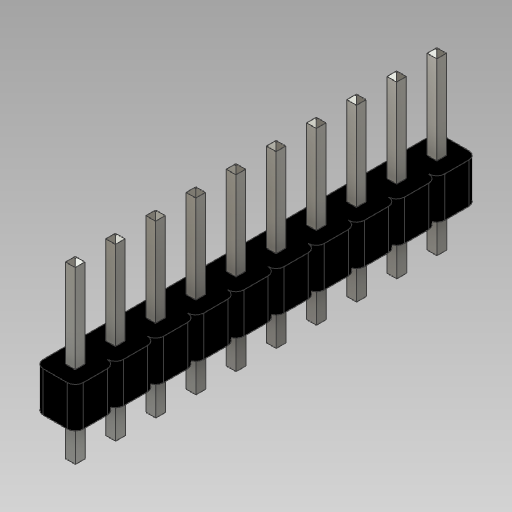
# Autodesk Inventor part: 10 pin header
Saved by Autodesk Inventor 2020 (Build 240168000, 168)
## iProperties
Created: 2017-07-30
Part Number: 10 pin header
Material: Generic
Document SubType Name: Modeling
Designer: Alex
Density: 1 g/cm^3
Appearance: Default
Author: Alex
Autodesk Inventor part; units mm, degrees
ref_plane "YZ Plane" through (0, 0, 0) normal (1, 0, 0) x (0, 1, 0)
ref_plane "XZ Plane" through (0, 0, 0) normal (0, 1, 0) x (-1, 0, 0)
ref_plane "XY Plane" through (0, 0, 0) normal (0, 0, 1) x (1, 0, 0)
sketch "Sketch1" plane through (0, 0, 0) normal (0, 1, 0) x (-1, 0, 0)
  line L0 (-0.762, -1.27) -> (0.762, -1.27)
  line L1 (1.27, -0.762) -> (1.27, 0.762)
  line L2 (0.762, 1.27) -> (-0.762, 1.27)
  line L3 (-1.27, 0.762) -> (-1.27, -0.762)
  line L4 (-1.27, -1.27) -> (1.27, 1.27) construction
  line L5 (1.27, -1.27) -> (-1.27, 1.27) construction
  arc A0 (1.27, 0.762) -> (0.762, 1.27) centre (0.762, 0.762) ccw
  arc A1 (0.762, -1.27) -> (1.27, -0.762) centre (0.762, -0.762) ccw
  arc A2 (-1.27, -0.762) -> (-0.762, -1.27) centre (-0.762, -0.762) ccw
  arc A3 (-0.762, 1.27) -> (-1.27, 0.762) centre (-0.762, 0.762) ccw
  line L6 (-0.762, -3.81) -> (0.762, -3.81)
  line L7 (1.27, -3.302) -> (1.27, -1.778)
  line L8 (0.762, -1.27) -> (-0.762, -1.27)
  line L9 (-1.27, -1.778) -> (-1.27, -3.302)
  line L10 (-1.27, -3.81) -> (1.27, -1.27) construction
  line L11 (1.27, -3.81) -> (-1.27, -1.27) construction
  arc A4 (1.27, -1.778) -> (0.762, -1.27) centre (0.762, -1.778) ccw
  arc A5 (0.762, -3.81) -> (1.27, -3.302) centre (0.762, -3.302) ccw
  arc A6 (-1.27, -3.302) -> (-0.762, -3.81) centre (-0.762, -3.302) ccw
  arc A7 (-0.762, -1.27) -> (-1.27, -1.778) centre (-0.762, -1.778) ccw
  line L12 (-0.762, -6.35) -> (0.762, -6.35)
  line L13 (1.27, -5.842) -> (1.27, -4.318)
  line L14 (0.762, -3.81) -> (-0.762, -3.81)
  line L15 (-1.27, -4.318) -> (-1.27, -5.842)
  line L16 (-1.27, -6.35) -> (1.27, -3.81) construction
  line L17 (1.27, -6.35) -> (-1.27, -3.81) construction
  arc A8 (1.27, -4.318) -> (0.762, -3.81) centre (0.762, -4.318) ccw
  arc A9 (0.762, -6.35) -> (1.27, -5.842) centre (0.762, -5.842) ccw
  arc A10 (-1.27, -5.842) -> (-0.762, -6.35) centre (-0.762, -5.842) ccw
  arc A11 (-0.762, -3.81) -> (-1.27, -4.318) centre (-0.762, -4.318) ccw
  line L18 (-0.762, -8.89) -> (0.762, -8.89)
  line L19 (1.27, -8.382) -> (1.27, -6.858)
  line L20 (0.762, -6.35) -> (-0.762, -6.35)
  line L21 (-1.27, -6.858) -> (-1.27, -8.382)
  line L22 (-1.27, -8.89) -> (1.27, -6.35) construction
  line L23 (1.27, -8.89) -> (-1.27, -6.35) construction
  arc A12 (1.27, -6.858) -> (0.762, -6.35) centre (0.762, -6.858) ccw
  arc A13 (0.762, -8.89) -> (1.27, -8.382) centre (0.762, -8.382) ccw
  arc A14 (-1.27, -8.382) -> (-0.762, -8.89) centre (-0.762, -8.382) ccw
  arc A15 (-0.762, -6.35) -> (-1.27, -6.858) centre (-0.762, -6.858) ccw
  line L24 (-0.762, -11.43) -> (0.762, -11.43)
  line L25 (1.27, -10.922) -> (1.27, -9.398)
  line L26 (0.762, -8.89) -> (-0.762, -8.89)
  line L27 (-1.27, -9.398) -> (-1.27, -10.922)
  line L28 (-1.27, -11.43) -> (1.27, -8.89) construction
  line L29 (1.27, -11.43) -> (-1.27, -8.89) construction
  arc A16 (1.27, -9.398) -> (0.762, -8.89) centre (0.762, -9.398) ccw
  arc A17 (0.762, -11.43) -> (1.27, -10.922) centre (0.762, -10.922) ccw
  arc A18 (-1.27, -10.922) -> (-0.762, -11.43) centre (-0.762, -10.922) ccw
  arc A19 (-0.762, -8.89) -> (-1.27, -9.398) centre (-0.762, -9.398) ccw
  line L30 (-0.762, -13.97) -> (0.762, -13.97)
  line L31 (1.27, -13.462) -> (1.27, -11.938)
  line L32 (0.762, -11.43) -> (-0.762, -11.43)
  line L33 (-1.27, -11.938) -> (-1.27, -13.462)
  line L34 (-1.27, -13.97) -> (1.27, -11.43) construction
  line L35 (1.27, -13.97) -> (-1.27, -11.43) construction
  arc A20 (1.27, -11.938) -> (0.762, -11.43) centre (0.762, -11.938) ccw
  arc A21 (0.762, -13.97) -> (1.27, -13.462) centre (0.762, -13.462) ccw
  arc A22 (-1.27, -13.462) -> (-0.762, -13.97) centre (-0.762, -13.462) ccw
  arc A23 (-0.762, -11.43) -> (-1.27, -11.938) centre (-0.762, -11.938) ccw
  line L36 (-0.762, -16.51) -> (0.762, -16.51)
  line L37 (1.27, -16.002) -> (1.27, -14.478)
  line L38 (0.762, -13.97) -> (-0.762, -13.97)
  line L39 (-1.27, -14.478) -> (-1.27, -16.002)
  line L40 (-1.27, -16.51) -> (1.27, -13.97) construction
  line L41 (1.27, -16.51) -> (-1.27, -13.97) construction
  arc A24 (1.27, -14.478) -> (0.762, -13.97) centre (0.762, -14.478) ccw
  arc A25 (0.762, -16.51) -> (1.27, -16.002) centre (0.762, -16.002) ccw
  arc A26 (-1.27, -16.002) -> (-0.762, -16.51) centre (-0.762, -16.002) ccw
  arc A27 (-0.762, -13.97) -> (-1.27, -14.478) centre (-0.762, -14.478) ccw
  line L42 (-0.762, -19.05) -> (0.762, -19.05)
  line L43 (1.27, -18.542) -> (1.27, -17.018)
  line L44 (0.762, -16.51) -> (-0.762, -16.51)
  line L45 (-1.27, -17.018) -> (-1.27, -18.542)
  line L46 (-1.27, -19.05) -> (1.27, -16.51) construction
  line L47 (1.27, -19.05) -> (-1.27, -16.51) construction
  arc A28 (1.27, -17.018) -> (0.762, -16.51) centre (0.762, -17.018) ccw
  arc A29 (0.762, -19.05) -> (1.27, -18.542) centre (0.762, -18.542) ccw
  arc A30 (-1.27, -18.542) -> (-0.762, -19.05) centre (-0.762, -18.542) ccw
  arc A31 (-0.762, -16.51) -> (-1.27, -17.018) centre (-0.762, -17.018) ccw
  line L48 (-0.762, -21.59) -> (0.762, -21.59)
  line L49 (1.27, -21.082) -> (1.27, -19.558)
  line L50 (0.762, -19.05) -> (-0.762, -19.05)
  line L51 (-1.27, -19.558) -> (-1.27, -21.082)
  line L52 (-1.27, -21.59) -> (1.27, -19.05) construction
  line L53 (1.27, -21.59) -> (-1.27, -19.05) construction
  arc A32 (1.27, -19.558) -> (0.762, -19.05) centre (0.762, -19.558) ccw
  arc A33 (0.762, -21.59) -> (1.27, -21.082) centre (0.762, -21.082) ccw
  arc A34 (-1.27, -21.082) -> (-0.762, -21.59) centre (-0.762, -21.082) ccw
  arc A35 (-0.762, -19.05) -> (-1.27, -19.558) centre (-0.762, -19.558) ccw
  line L54 (-0.762, -24.13) -> (0.762, -24.13)
  line L55 (1.27, -23.622) -> (1.27, -22.098)
  line L56 (0.762, -21.59) -> (-0.762, -21.59)
  line L57 (-1.27, -22.098) -> (-1.27, -23.622)
  line L58 (-1.27, -24.13) -> (1.27, -21.59) construction
  line L59 (1.27, -24.13) -> (-1.27, -21.59) construction
  arc A36 (1.27, -22.098) -> (0.762, -21.59) centre (0.762, -22.098) ccw
  arc A37 (0.762, -24.13) -> (1.27, -23.622) centre (0.762, -23.622) ccw
  arc A38 (-1.27, -23.622) -> (-0.762, -24.13) centre (-0.762, -23.622) ccw
  arc A39 (-0.762, -21.59) -> (-1.27, -22.098) centre (-0.762, -22.098) ccw
  line L60 (-0.762, -26.67) -> (0.762, -26.67)
  line L61 (1.27, -26.162) -> (1.27, -24.638)
  line L62 (0.762, -24.13) -> (-0.762, -24.13)
  line L63 (-1.27, -24.638) -> (-1.27, -26.162)
  line L64 (-1.27, -26.67) -> (1.27, -24.13) construction
  line L65 (1.27, -26.67) -> (-1.27, -24.13) construction
  arc A40 (1.27, -24.638) -> (0.762, -24.13) centre (0.762, -24.638) ccw
  arc A41 (0.762, -26.67) -> (1.27, -26.162) centre (0.762, -26.162) ccw
  arc A42 (-1.27, -26.162) -> (-0.762, -26.67) centre (-0.762, -26.162) ccw
  arc A43 (-0.762, -24.13) -> (-1.27, -24.638) centre (-0.762, -24.638) ccw
  line L66 (-0.762, -29.21) -> (0.762, -29.21)
  line L67 (1.27, -28.702) -> (1.27, -27.178)
  line L68 (0.762, -26.67) -> (-0.762, -26.67)
  line L69 (-1.27, -27.178) -> (-1.27, -28.702)
  line L70 (-1.27, -29.21) -> (1.27, -26.67) construction
  line L71 (1.27, -29.21) -> (-1.27, -26.67) construction
  arc A44 (1.27, -27.178) -> (0.762, -26.67) centre (0.762, -27.178) ccw
  arc A45 (0.762, -29.21) -> (1.27, -28.702) centre (0.762, -28.702) ccw
  arc A46 (-1.27, -28.702) -> (-0.762, -29.21) centre (-0.762, -28.702) ccw
  arc A47 (-0.762, -26.67) -> (-1.27, -27.178) centre (-0.762, -27.178) ccw
  line L72 (-0.762, -31.75) -> (0.762, -31.75)
  line L73 (1.27, -31.242) -> (1.27, -29.718)
  line L74 (0.762, -29.21) -> (-0.762, -29.21)
  line L75 (-1.27, -29.718) -> (-1.27, -31.242)
  line L76 (-1.27, -31.75) -> (1.27, -29.21) construction
  line L77 (1.27, -31.75) -> (-1.27, -29.21) construction
  arc A48 (1.27, -29.718) -> (0.762, -29.21) centre (0.762, -29.718) ccw
  arc A49 (0.762, -31.75) -> (1.27, -31.242) centre (0.762, -31.242) ccw
  arc A50 (-1.27, -31.242) -> (-0.762, -31.75) centre (-0.762, -31.242) ccw
  arc A51 (-0.762, -29.21) -> (-1.27, -29.718) centre (-0.762, -29.718) ccw
  line L78 (-0.762, -34.29) -> (0.762, -34.29)
  line L79 (1.27, -33.782) -> (1.27, -32.258)
  line L80 (0.762, -31.75) -> (-0.762, -31.75)
  line L81 (-1.27, -32.258) -> (-1.27, -33.782)
  line L82 (-1.27, -34.29) -> (1.27, -31.75) construction
  line L83 (1.27, -34.29) -> (-1.27, -31.75) construction
  arc A52 (1.27, -32.258) -> (0.762, -31.75) centre (0.762, -32.258) ccw
  arc A53 (0.762, -34.29) -> (1.27, -33.782) centre (0.762, -33.782) ccw
  arc A54 (-1.27, -33.782) -> (-0.762, -34.29) centre (-0.762, -33.782) ccw
  arc A55 (-0.762, -31.75) -> (-1.27, -32.258) centre (-0.762, -32.258) ccw
  line L84 (-0.762, -36.83) -> (0.762, -36.83)
  line L85 (1.27, -36.322) -> (1.27, -34.798)
  line L86 (0.762, -34.29) -> (-0.762, -34.29)
  line L87 (-1.27, -34.798) -> (-1.27, -36.322)
  line L88 (-1.27, -36.83) -> (1.27, -34.29) construction
  line L89 (1.27, -36.83) -> (-1.27, -34.29) construction
  arc A56 (1.27, -34.798) -> (0.762, -34.29) centre (0.762, -34.798) ccw
  arc A57 (0.762, -36.83) -> (1.27, -36.322) centre (0.762, -36.322) ccw
  arc A58 (-1.27, -36.322) -> (-0.762, -36.83) centre (-0.762, -36.322) ccw
  arc A59 (-0.762, -34.29) -> (-1.27, -34.798) centre (-0.762, -34.798) ccw
  line L90 (-0.762, -39.37) -> (0.762, -39.37)
  line L91 (1.27, -38.862) -> (1.27, -37.338)
  line L92 (0.762, -36.83) -> (-0.762, -36.83)
  line L93 (-1.27, -37.338) -> (-1.27, -38.862)
  line L94 (-1.27, -39.37) -> (1.27, -36.83) construction
  line L95 (1.27, -39.37) -> (-1.27, -36.83) construction
  arc A60 (1.27, -37.338) -> (0.762, -36.83) centre (0.762, -37.338) ccw
  arc A61 (0.762, -39.37) -> (1.27, -38.862) centre (0.762, -38.862) ccw
  arc A62 (-1.27, -38.862) -> (-0.762, -39.37) centre (-0.762, -38.862) ccw
  arc A63 (-0.762, -36.83) -> (-1.27, -37.338) centre (-0.762, -37.338) ccw
  point P0 (0, 0)
  point P1 (0, -2.54)
  point P2 (0, -5.08)
  point P3 (0, -7.62)
  point P4 (0, -10.16)
  point P5 (0, -12.7)
  point P6 (0, -15.24)
  point P7 (0, -17.78)
  point P8 (0, -20.32)
  point P9 (0, -22.86)
  point P10 (0, -25.4)
  point P11 (0, -27.94)
  point P12 (0, -30.48)
  point P13 (0, -33.02)
  point P14 (0, -35.56)
  point P15 (0, -38.1)
  dimension "d0" = 2.54
  dimension "d1" = 0.508
  dimension "d4" = 2.54
  constraints: 192 end point, 128 point on circle, 128 point on line, 64 centre point, 32 midpoint, 8 tangent, 3 equal radius, 2 parallel, 2 perpendicular, 1 collinear, 1 horizontal, 1 vertical, 404 other
  measures "d0" distance between parallel lines of L0 L2
  measures "d1" radius of A0
  measures "d4" distance of point (0, 0) point (0, -2.54)
extrude "Extrusion1" add sketch "Sketch1" along normal mid plane 2.54
sketch "Sketch2" plane through (0, 1.27, 0) normal (0, 1, 0) x (1, 0, 0)
  line L0 (-0.3048, 0.3048) -> (0.3048, 0.3048)
  line L1 (0.3048, 0.3048) -> (0.3048, -0.3048)
  line L2 (0.3048, -0.3048) -> (-0.3048, -0.3048)
  line L3 (-0.3048, -0.3048) -> (-0.3048, 0.3048)
  line L4 (-0.3048, 0.3048) -> (0.3048, -0.3048) construction
  line L5 (0.3048, 0.3048) -> (-0.3048, -0.3048) construction
  line L6 (-1.27, 0.762) -> (-1.27, -0.762) projected
  line L7 (-0.3048, 2.8448) -> (0.3048, 2.8448)
  line L8 (0.3048, 2.8448) -> (0.3048, 2.2352)
  line L9 (0.3048, 2.2352) -> (-0.3048, 2.2352)
  line L10 (-0.3048, 2.2352) -> (-0.3048, 2.8448)
  line L11 (-0.3048, 2.8448) -> (0.3048, 2.2352) construction
  line L12 (0.3048, 2.8448) -> (-0.3048, 2.2352) construction
  line L13 (-0.3048, 5.3848) -> (0.3048, 5.3848)
  line L14 (0.3048, 5.3848) -> (0.3048, 4.7752)
  line L15 (0.3048, 4.7752) -> (-0.3048, 4.7752)
  line L16 (-0.3048, 4.7752) -> (-0.3048, 5.3848)
  line L17 (-0.3048, 5.3848) -> (0.3048, 4.7752) construction
  line L18 (0.3048, 5.3848) -> (-0.3048, 4.7752) construction
  line L19 (-0.3048, 7.9248) -> (0.3048, 7.9248)
  line L20 (0.3048, 7.9248) -> (0.3048, 7.3152)
  line L21 (0.3048, 7.3152) -> (-0.3048, 7.3152)
  line L22 (-0.3048, 7.3152) -> (-0.3048, 7.9248)
  line L23 (-0.3048, 7.9248) -> (0.3048, 7.3152) construction
  line L24 (0.3048, 7.9248) -> (-0.3048, 7.3152) construction
  line L25 (-0.3048, 10.4648) -> (0.3048, 10.4648)
  line L26 (0.3048, 10.4648) -> (0.3048, 9.8552)
  line L27 (0.3048, 9.8552) -> (-0.3048, 9.8552)
  line L28 (-0.3048, 9.8552) -> (-0.3048, 10.4648)
  line L29 (-0.3048, 10.4648) -> (0.3048, 9.8552) construction
  line L30 (0.3048, 10.4648) -> (-0.3048, 9.8552) construction
  line L31 (-0.3048, 13.0048) -> (0.3048, 13.0048)
  line L32 (0.3048, 13.0048) -> (0.3048, 12.3952)
  line L33 (0.3048, 12.3952) -> (-0.3048, 12.3952)
  line L34 (-0.3048, 12.3952) -> (-0.3048, 13.0048)
  line L35 (-0.3048, 13.0048) -> (0.3048, 12.3952) construction
  line L36 (0.3048, 13.0048) -> (-0.3048, 12.3952) construction
  line L37 (-0.3048, 15.5448) -> (0.3048, 15.5448)
  line L38 (0.3048, 15.5448) -> (0.3048, 14.9352)
  line L39 (0.3048, 14.9352) -> (-0.3048, 14.9352)
  line L40 (-0.3048, 14.9352) -> (-0.3048, 15.5448)
  line L41 (-0.3048, 15.5448) -> (0.3048, 14.9352) construction
  line L42 (0.3048, 15.5448) -> (-0.3048, 14.9352) construction
  line L43 (-0.3048, 18.0848) -> (0.3048, 18.0848)
  line L44 (0.3048, 18.0848) -> (0.3048, 17.4752)
  line L45 (0.3048, 17.4752) -> (-0.3048, 17.4752)
  line L46 (-0.3048, 17.4752) -> (-0.3048, 18.0848)
  line L47 (-0.3048, 18.0848) -> (0.3048, 17.4752) construction
  line L48 (0.3048, 18.0848) -> (-0.3048, 17.4752) construction
  line L49 (-0.3048, 20.6248) -> (0.3048, 20.6248)
  line L50 (0.3048, 20.6248) -> (0.3048, 20.0152)
  line L51 (0.3048, 20.0152) -> (-0.3048, 20.0152)
  line L52 (-0.3048, 20.0152) -> (-0.3048, 20.6248)
  line L53 (-0.3048, 20.6248) -> (0.3048, 20.0152) construction
  line L54 (0.3048, 20.6248) -> (-0.3048, 20.0152) construction
  line L55 (-0.3048, 23.1648) -> (0.3048, 23.1648)
  line L56 (0.3048, 23.1648) -> (0.3048, 22.5552)
  line L57 (0.3048, 22.5552) -> (-0.3048, 22.5552)
  line L58 (-0.3048, 22.5552) -> (-0.3048, 23.1648)
  line L59 (-0.3048, 23.1648) -> (0.3048, 22.5552) construction
  line L60 (0.3048, 23.1648) -> (-0.3048, 22.5552) construction
  line L61 (-0.3048, 25.7048) -> (0.3048, 25.7048)
  line L62 (0.3048, 25.7048) -> (0.3048, 25.0952)
  line L63 (0.3048, 25.0952) -> (-0.3048, 25.0952)
  line L64 (-0.3048, 25.0952) -> (-0.3048, 25.7048)
  line L65 (-0.3048, 25.7048) -> (0.3048, 25.0952) construction
  line L66 (0.3048, 25.7048) -> (-0.3048, 25.0952) construction
  line L67 (-0.3048, 28.2448) -> (0.3048, 28.2448)
  line L68 (0.3048, 28.2448) -> (0.3048, 27.6352)
  line L69 (0.3048, 27.6352) -> (-0.3048, 27.6352)
  line L70 (-0.3048, 27.6352) -> (-0.3048, 28.2448)
  line L71 (-0.3048, 28.2448) -> (0.3048, 27.6352) construction
  line L72 (0.3048, 28.2448) -> (-0.3048, 27.6352) construction
  line L73 (-0.3048, 30.7848) -> (0.3048, 30.7848)
  line L74 (0.3048, 30.7848) -> (0.3048, 30.1752)
  line L75 (0.3048, 30.1752) -> (-0.3048, 30.1752)
  line L76 (-0.3048, 30.1752) -> (-0.3048, 30.7848)
  line L77 (-0.3048, 30.7848) -> (0.3048, 30.1752) construction
  line L78 (0.3048, 30.7848) -> (-0.3048, 30.1752) construction
  line L79 (-0.3048, 33.3248) -> (0.3048, 33.3248)
  line L80 (0.3048, 33.3248) -> (0.3048, 32.7152)
  line L81 (0.3048, 32.7152) -> (-0.3048, 32.7152)
  line L82 (-0.3048, 32.7152) -> (-0.3048, 33.3248)
  line L83 (-0.3048, 33.3248) -> (0.3048, 32.7152) construction
  line L84 (0.3048, 33.3248) -> (-0.3048, 32.7152) construction
  line L85 (-0.3048, 35.8648) -> (0.3048, 35.8648)
  line L86 (0.3048, 35.8648) -> (0.3048, 35.2552)
  line L87 (0.3048, 35.2552) -> (-0.3048, 35.2552)
  line L88 (-0.3048, 35.2552) -> (-0.3048, 35.8648)
  line L89 (-0.3048, 35.8648) -> (0.3048, 35.2552) construction
  line L90 (0.3048, 35.8648) -> (-0.3048, 35.2552) construction
  line L91 (-0.3048, 38.4048) -> (0.3048, 38.4048)
  line L92 (0.3048, 38.4048) -> (0.3048, 37.7952)
  line L93 (0.3048, 37.7952) -> (-0.3048, 37.7952)
  line L94 (-0.3048, 37.7952) -> (-0.3048, 38.4048)
  line L95 (-0.3048, 38.4048) -> (0.3048, 37.7952) construction
  line L96 (0.3048, 38.4048) -> (-0.3048, 37.7952) construction
  point P0 (0, 0)
  dimension "d11" = 0.6096
  dimension "d14" = 2.54
  constraints: 192 end point, 2 midpoint, 2 parallel, 2 perpendicular, 1 horizontal, 1 vertical, 150 other
  measures "d11" distance of L2.end L0.start
  measures "d14" distance of L0.start L7.start
extrude "Extrusion2" add sketch "Sketch2" along normal blind 5.842
chamfer "Chamfer2" distance 0.254 angle 45 64 edges at (0, 7.112, -20.6248) (-0.3048, 7.112, -20.32) (0.3048, 7.112, -20.32) (0, 7.112, -20.0152) (0, 7.112, -18.0848) (-0.3048, 7.112, -17.78) (0, 7.112, -17.4752) (0.3048, 7.112, -17.78) (0, 7.112, -15.5448) (-0.3048, 7.112, -15.24) (0.3048, 7.112, -15.24) (0, 7.112, -13.0048) (-0.3048, 7.112, -12.7) (0, 7.112, -12.3952) (0.3048, 7.112, -12.7) (0, 7.112, -14.9352) (-0.3048, 7.112, -7.62) (0, 7.112, -7.3152) (0.3048, 7.112, -7.62) (0, 7.112, -9.8552) (0, 7.112, -10.4648) (-0.3048, 7.112, -10.16) (0.3048, 7.112, -10.16) (0, 7.112, -7.9248) (0, 7.112, -2.8448) (-0.3048, 7.112, -2.54) (0, 7.112, -2.2352) (0.3048, 7.112, -2.54) (0, 7.112, -4.7752) (0.3048, 7.112, -5.08) (0, 7.112, -5.3848) (-0.3048, 7.112, -5.08) (0, 7.112, -0.3048) (-0.3048, 7.112, 0) (0, 7.112, 0.3048) (0.3048, 7.112, 0) (0, 7.112, -23.1648) (-0.3048, 7.112, -22.86) (0, 7.112, -22.5552) (0.3048, 7.112, -22.86) (0, 7.112, -25.0952) (-0.3048, 7.112, -25.4) (0, 7.112, -25.7048) (0.3048, 7.112, -25.4) (0, 7.112, -28.2448) (0, 7.112, -27.6352) (0.3048, 7.112, -27.94) (-0.3048, 7.112, -27.94) (0.3048, 7.112, -30.48) (0, 7.112, -38.4048) (-0.3048, 7.112, -38.1) (0, 7.112, -37.7952) (0.3048, 7.112, -38.1) (0, 7.112, -35.8648) (-0.3048, 7.112, -35.56) (0, 7.112, -35.2552) (0.3048, 7.112, -35.56) (0, 7.112, -33.3248) (-0.3048, 7.112, -33.02) (0, 7.112, -32.7152) (0, 7.112, -30.1752) (0, 7.112, -30.7848) (-0.3048, 7.112, -30.48) (0.3048, 7.112, -33.02)
sketch "Sketch6" plane through (0, -1.27, 0) normal (0, -1, 0) x (1, 0, 0)
  line L0 (-0.3048, 0.3048) -> (-0.3048, -0.3048) projected
  line L1 (0.3175, -0.3175) -> (-0.3048, -0.3175)
  line L2 (-0.3048, -0.3175) -> (-0.3048, 0.3048)
  line L3 (-0.3048, 0.3048) -> (0.3175, 0.3048)
  line L4 (0.3175, 0.3048) -> (0.3175, -0.3175)
  line L5 (0.3175, -0.3175) -> (-0.3048, 0.3048) construction
  line L6 (-0.3048, -0.3175) -> (0.3175, 0.3048) construction
  line L7 (1.27, -0.762) -> (1.27, 0.762) construction
  line L8 (0.3175, -2.8575) -> (-0.3048, -2.8575)
  line L9 (-0.3048, -2.8575) -> (-0.3048, -2.2352)
  line L10 (-0.3048, -2.2352) -> (0.3175, -2.2352)
  line L11 (0.3175, -2.2352) -> (0.3175, -2.8575)
  line L12 (0.3175, -2.8575) -> (-0.3048, -2.2352) construction
  line L13 (-0.3048, -2.8575) -> (0.3175, -2.2352) construction
  line L14 (0.3175, -5.3975) -> (-0.3048, -5.3975)
  line L15 (-0.3048, -5.3975) -> (-0.3048, -4.7752)
  line L16 (-0.3048, -4.7752) -> (0.3175, -4.7752)
  line L17 (0.3175, -4.7752) -> (0.3175, -5.3975)
  line L18 (0.3175, -5.3975) -> (-0.3048, -4.7752) construction
  line L19 (-0.3048, -5.3975) -> (0.3175, -4.7752) construction
  line L20 (0.3175, -7.9375) -> (-0.3048, -7.9375)
  line L21 (-0.3048, -7.9375) -> (-0.3048, -7.3152)
  line L22 (-0.3048, -7.3152) -> (0.3175, -7.3152)
  line L23 (0.3175, -7.3152) -> (0.3175, -7.9375)
  line L24 (0.3175, -7.9375) -> (-0.3048, -7.3152) construction
  line L25 (-0.3048, -7.9375) -> (0.3175, -7.3152) construction
  line L26 (0.3175, -10.4775) -> (-0.3048, -10.4775)
  line L27 (-0.3048, -10.4775) -> (-0.3048, -9.8552)
  line L28 (-0.3048, -9.8552) -> (0.3175, -9.8552)
  line L29 (0.3175, -9.8552) -> (0.3175, -10.4775)
  line L30 (0.3175, -10.4775) -> (-0.3048, -9.8552) construction
  line L31 (-0.3048, -10.4775) -> (0.3175, -9.8552) construction
  line L32 (0.3175, -13.0175) -> (-0.3048, -13.0175)
  line L33 (-0.3048, -13.0175) -> (-0.3048, -12.3952)
  line L34 (-0.3048, -12.3952) -> (0.3175, -12.3952)
  line L35 (0.3175, -12.3952) -> (0.3175, -13.0175)
  line L36 (0.3175, -13.0175) -> (-0.3048, -12.3952) construction
  line L37 (-0.3048, -13.0175) -> (0.3175, -12.3952) construction
  line L38 (0.3175, -15.5575) -> (-0.3048, -15.5575)
  line L39 (-0.3048, -15.5575) -> (-0.3048, -14.9352)
  line L40 (-0.3048, -14.9352) -> (0.3175, -14.9352)
  line L41 (0.3175, -14.9352) -> (0.3175, -15.5575)
  line L42 (0.3175, -15.5575) -> (-0.3048, -14.9352) construction
  line L43 (-0.3048, -15.5575) -> (0.3175, -14.9352) construction
  line L44 (0.3175, -18.0975) -> (-0.3048, -18.0975)
  line L45 (-0.3048, -18.0975) -> (-0.3048, -17.4752)
  line L46 (-0.3048, -17.4752) -> (0.3175, -17.4752)
  line L47 (0.3175, -17.4752) -> (0.3175, -18.0975)
  line L48 (0.3175, -18.0975) -> (-0.3048, -17.4752) construction
  line L49 (-0.3048, -18.0975) -> (0.3175, -17.4752) construction
  line L50 (0.3175, -20.6375) -> (-0.3048, -20.6375)
  line L51 (-0.3048, -20.6375) -> (-0.3048, -20.0152)
  line L52 (-0.3048, -20.0152) -> (0.3175, -20.0152)
  line L53 (0.3175, -20.0152) -> (0.3175, -20.6375)
  line L54 (0.3175, -20.6375) -> (-0.3048, -20.0152) construction
  line L55 (-0.3048, -20.6375) -> (0.3175, -20.0152) construction
  line L56 (0.3175, -23.1775) -> (-0.3048, -23.1775)
  line L57 (-0.3048, -23.1775) -> (-0.3048, -22.5552)
  line L58 (-0.3048, -22.5552) -> (0.3175, -22.5552)
  line L59 (0.3175, -22.5552) -> (0.3175, -23.1775)
  line L60 (0.3175, -23.1775) -> (-0.3048, -22.5552) construction
  line L61 (-0.3048, -23.1775) -> (0.3175, -22.5552) construction
  line L62 (0.3175, -25.7175) -> (-0.3048, -25.7175)
  line L63 (-0.3048, -25.7175) -> (-0.3048, -25.0952)
  line L64 (-0.3048, -25.0952) -> (0.3175, -25.0952)
  line L65 (0.3175, -25.0952) -> (0.3175, -25.7175)
  line L66 (0.3175, -25.7175) -> (-0.3048, -25.0952) construction
  line L67 (-0.3048, -25.7175) -> (0.3175, -25.0952) construction
  line L68 (0.3175, -28.2575) -> (-0.3048, -28.2575)
  line L69 (-0.3048, -28.2575) -> (-0.3048, -27.6352)
  line L70 (-0.3048, -27.6352) -> (0.3175, -27.6352)
  line L71 (0.3175, -27.6352) -> (0.3175, -28.2575)
  line L72 (0.3175, -28.2575) -> (-0.3048, -27.6352) construction
  line L73 (-0.3048, -28.2575) -> (0.3175, -27.6352) construction
  line L74 (0.3175, -30.7975) -> (-0.3048, -30.7975)
  line L75 (-0.3048, -30.7975) -> (-0.3048, -30.1752)
  line L76 (-0.3048, -30.1752) -> (0.3175, -30.1752)
  line L77 (0.3175, -30.1752) -> (0.3175, -30.7975)
  line L78 (0.3175, -30.7975) -> (-0.3048, -30.1752) construction
  line L79 (-0.3048, -30.7975) -> (0.3175, -30.1752) construction
  line L80 (0.3175, -33.3375) -> (-0.3048, -33.3375)
  line L81 (-0.3048, -33.3375) -> (-0.3048, -32.7152)
  line L82 (-0.3048, -32.7152) -> (0.3175, -32.7152)
  line L83 (0.3175, -32.7152) -> (0.3175, -33.3375)
  line L84 (0.3175, -33.3375) -> (-0.3048, -32.7152) construction
  line L85 (-0.3048, -33.3375) -> (0.3175, -32.7152) construction
  line L86 (0.3175, -35.8775) -> (-0.3048, -35.8775)
  line L87 (-0.3048, -35.8775) -> (-0.3048, -35.2552)
  line L88 (-0.3048, -35.2552) -> (0.3175, -35.2552)
  line L89 (0.3175, -35.2552) -> (0.3175, -35.8775)
  line L90 (0.3175, -35.8775) -> (-0.3048, -35.2552) construction
  line L91 (-0.3048, -35.8775) -> (0.3175, -35.2552) construction
  line L92 (0.3175, -38.4175) -> (-0.3048, -38.4175)
  line L93 (-0.3048, -38.4175) -> (-0.3048, -37.7952)
  line L94 (-0.3048, -37.7952) -> (0.3175, -37.7952)
  line L95 (0.3175, -37.7952) -> (0.3175, -38.4175)
  line L96 (0.3175, -38.4175) -> (-0.3048, -37.7952) construction
  line L97 (-0.3048, -38.4175) -> (0.3175, -37.7952) construction
  point P0 (0.0064, -0.0063)
  point P1 (-0.3048, -2.8448)
  point P2 (0.0064, -2.5463)
  point P3 (-0.3048, -5.3848)
  point P4 (0.0064, -5.0863)
  point P5 (-0.3048, -7.9248)
  point P6 (0.0064, -7.6263)
  point P7 (-0.3048, -10.4648)
  point P8 (0.0064, -10.1663)
  point P9 (-0.3048, -13.0048)
  point P10 (0.0064, -12.7064)
  point P11 (-0.3048, -15.5448)
  point P12 (0.0064, -15.2463)
  point P13 (-0.3048, -18.0848)
  point P14 (0.0064, -17.7863)
  point P15 (-0.3048, -20.6248)
  point P16 (0.0064, -20.3263)
  point P17 (-0.3048, -23.1648)
  point P18 (0.0064, -22.8664)
  point P19 (-0.3048, -25.7048)
  point P20 (0.0064, -25.4063)
  point P21 (-0.3048, -28.2448)
  point P22 (0.0064, -27.9463)
  point P23 (-0.3048, -30.7848)
  point P24 (0.0064, -30.4864)
  point P25 (-0.3048, -33.3248)
  point P26 (0.0064, -33.0264)
  point P27 (-0.3048, -35.8648)
  point P28 (0.0064, -35.5663)
  point P29 (-0.3048, -38.4048)
  point P30 (0.0064, -38.1063)
  dimension "d31" = 2.54
  constraints: 192 end point, 32 midpoint, 2 parallel, 1 horizontal, 1 perpendicular, 1 vertical, 180 other
  measures "d31" distance of L1.start L8.start
extrude "Extrusion3" add sketch "Sketch6" along normal blind 2.8956
chamfer "Chamfer4" distance 0.254 angle 45 64 edges at (0.0063, -4.1656, -18.0975) (0.0064, -4.1656, -17.4752) (-0.3048, -4.1656, -17.7863) (0.3175, -4.1656, -17.7863) (0.3175, -4.1656, -15.2463) (0.0064, -4.1656, -14.9352) (-0.3048, -4.1656, -15.2463) (0.0063, -4.1656, -15.5575) (0.0063, -4.1656, -23.1775) (0.3175, -4.1656, -22.8664) (0.0064, -4.1656, -22.5552) (-0.3048, -4.1656, -22.8664) (0.0063, -4.1656, -25.7175) (0.3175, -4.1656, -25.4064) (-0.3048, -4.1656, -25.4063) (0.0064, -4.1656, -25.0952) (0.0063, -4.1656, -28.2575) (0.3175, -4.1656, -27.9464) (0.0064, -4.1656, -27.6352) (-0.3048, -4.1656, -27.9463) (0.0063, -4.1656, -20.6375) (0.3175, -4.1656, -20.3264) (0.0064, -4.1656, -20.0152) (-0.3048, -4.1656, -20.3263) (0.0063, -4.1656, -30.7975) (0.3175, -4.1656, -30.4864) (-0.3048, -4.1656, -30.4864) (0.0064, -4.1656, -30.1752) (0.0063, -4.1656, -33.3375) (0.0064, -4.1656, -32.7152) (-0.3048, -4.1656, -33.0264) (0.3175, -4.1656, -33.0264) (0.0064, -4.1656, -35.2552) (0.3175, -4.1656, -35.5663) (-0.3048, -4.1656, -35.5663) (0.0063, -4.1656, -35.8775) (0.0063, -4.1656, -38.4175) (0.3175, -4.1656, -38.1064) (0.0064, -4.1656, -37.7952) (-0.3048, -4.1656, -38.1063) (0.0063, -4.1656, -13.0175) (0.3175, -4.1656, -12.7064) (0.0064, -4.1656, -12.3952) (-0.3048, -4.1656, -12.7064) (0.0063, -4.1656, -10.4775) (0.3175, -4.1656, -10.1663) (-0.3048, -4.1656, -10.1663) (0.0064, -4.1656, -9.8552) (0.0063, -4.1656, -7.9375) (0.3175, -4.1656, -7.6263) (0.0064, -4.1656, -7.3152) (-0.3048, -4.1656, -7.6263) (0.0063, -4.1656, -2.8575) (0.3175, -4.1656, -2.5463) (0.0064, -4.1656, -2.2352) (-0.3048, -4.1656, -2.5463) (0.0064, -4.1656, -4.7752) (0.3175, -4.1656, -5.0863) (0.0063, -4.1656, -5.3975) (-0.3048, -4.1656, -5.0863) (0.0063, -4.1656, -0.3175) (0.3175, -4.1656, -0.0063) (0.0064, -4.1656, 0.3048) (-0.3048, -4.1656, -0.0063)
sketch "Sketch9" plane through (1.27, -1.27, -0.762) normal (1, 0, 0) x (0, 0, -1)
  line L0 (0.508, 0) -> (0.508, 2.54) projected
  line L1 (13.208, -3.2078) -> (-3.6811, -3.2078)
  line L2 (-3.6811, -3.2078) -> (-3.6811, 9.934)
  line L3 (-3.6811, 9.934) -> (13.208, 9.934)
  line L4 (13.208, 9.934) -> (13.208, -3.2078)
  line L5 (13.208, 0) -> (13.208, 2.54) projected
  point P0 (-0.762, 1.27)
  constraints: 8 end point, 2 parallel, 1 horizontal, 1 perpendicular, 1 point on line
extrude "Extrusion4" cut sketch "Sketch9" against normal through all
body "Solid1"
